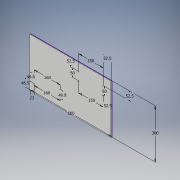
# Autodesk Inventor part: mounting plate
Saved by Autodesk Inventor 2019 (Build 230136000, 136)
## iProperties
Created: 2020-11-04
Part Number: mounting plate
Material: Generic
Document SubType Name: Modeling
Designer: 6raby
Density: 1 g/cm^3
Appearance: Default
Author: 6raby
Autodesk Inventor part; units mm, degrees
ref_plane "YZ Plane" through (0, 0, 0) normal (1, 0, 0) x (0, 1, 0)
ref_plane "XZ Plane" through (0, 0, 0) normal (0, 1, 0) x (-1, 0, 0)
ref_plane "XY Plane" through (0, 0, 0) normal (0, 0, 1) x (1, 0, 0)
sketch "Sketch1" plane through (0, 0, 0) normal (0, 0, 1) x (1, 0, 0)
  line L0 (0, 0) -> (500, 0)
  line L1 (500, 0) -> (500, 300)
  line L2 (500, 300) -> (0, 300)
  line L3 (0, 300) -> (0, 0)
  point P0 (23, 46.5)
  point P1 (23, 96.3)
  point P2 (183, 46.5)
  point P3 (183, 96.3)
  point P4 (447.5, 247.5)
  point P5 (297.5, 247.5)
  point P6 (297.5, 197.5)
  point P7 (447.5, 197.5)
  dimension "d0" = 500
  dimension "d1" = 300
  dimension "d2" = 46.5
  dimension "d3" = 23
  dimension "d4" = 49.8
  dimension "d5" = 160
  dimension "d6" = 160
  dimension "d7" = 49.8
  dimension "d8" = 52.5
  dimension "d9" = 52.5
  dimension "d11" = 150
  dimension "d12" = 52.5
  dimension "d13" = 150
  dimension "d14" = 50
  dimension "d15" = 50
  dimension "d16" = 52.5
  constraints: 8 end point, 2 perpendicular, 1 horizontal, 1 vertical
  measures "d0" distance of L0.start L0.end
  measures "d1" distance of L0.end L1.end
  measures "d2" vertical distance of point (23, 46.5) L0.start
  measures "d3" horizontal distance of point (23, 46.5) L0.start
  measures "d4" distance of point (23, 96.3) point (23, 46.5)
  measures "d5" distance of point (183, 46.5) point (23, 46.5)
  measures "d6" distance of point (23, 96.3) point (183, 96.3)
  measures "d7" distance of point (183, 46.5) point (183, 96.3)
  measures "d8" horizontal distance of point (447.5, 247.5) L1.end
  measures "d9" horizontal distance of point (447.5, 247.5) L1.end
  measures "d11" distance of point (447.5, 247.5) point (297.5, 247.5)
  measures "d12" distance from line of L1 point (447.5, 197.5)
  measures "d13" distance of point (447.5, 197.5) point (297.5, 197.5)
  measures "d14" distance of point (297.5, 247.5) point (297.5, 197.5)
  measures "d15" distance of point (447.5, 197.5) point (447.5, 247.5)
  measures "d16" distance from line of L2 point (297.5, 247.5)
extrude "Extrusion1" add sketch "Sketch1" along normal blind 5
hole "Hole1" at (297.5, 197.5, 0) at (297.5, 247.5, 0) at (447.5, 247.5, 0) at (447.5, 197.5, 0) direction (0, 0, 1) diameter 3 end through all
hole "Hole2" at (23, 46.5, 0) at (23, 96.3, 0) at (183, 46.5, 0) at (183, 96.3, 0) direction (0, 0, 1) diameter 2.5 end through all
body "Solid1"
